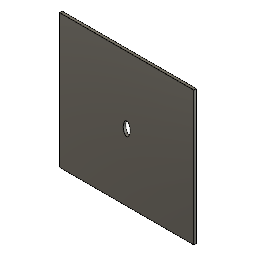
Table_17p1_Problem_9 (Autodesk Fusion 360 design; units mm, degrees)
Autodesk Fusion 360 part; units mm, degrees
sketch "Sketch1" plane through (0, 0, 0) normal (0, 0, 1) x (1, 0, 0)
  line L0 (-250, 250) -> (250, 250)
  line L1 (250, 250) -> (250, -250)
  line L2 (250, -250) -> (-250, -250)
  line L3 (-250, -250) -> (-250, 250)
  line L4 (0, 250) -> (0, -250) construction
  line L5 (-250, 0) -> (250, 0) construction
  ellipse E0 centre (0, 0) end of major axis (0, 25) minor radius 12.5
  line L6 (0, -25) -> (0, 25)
  line L7 (12.5, 0) -> (-12.5, 0)
  dimension "Total_Width" = 500
  dimension "Major_Radius" = 25
  dimension "Minor_Radius" = 12.5
  constraint horizontal L0
  constraint vertical L1
  constraint horizontal L2
  constraint vertical L3
  constraint midpoint L0 L4.start
  constraint midpoint L2 L4.end
  constraint midpoint L3 L5.start
  constraint midpoint L1 L5.end
  constraint coincident E0.centre origin
  constraint coincident L5 E0.centre
  constraint coincident L4 E0.centre
  constraint equal L0 L1
  constraint perpendicular L5 L6
  constraint coincident E0 L6.start
  constraint coincident E0 L6.end
  constraint coincident E0 L7.start
  constraint coincident E0 L7.end
  measures "Total_Width" distance of L0.start L2.end
  measures "Major_Radius" distance of E0
extrude "Extrude1" add sketch "Sketch1" along normal mid plane 10
equation "Thickness = 1 cm"
